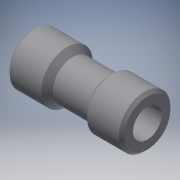
# Autodesk Inventor part: motor_coupling
Saved by Autodesk Inventor 2016 (Build 200138000, 138)
## iProperties
Created: 2016-12-23
Part Number: motor_coupling
Material: Generic
Document SubType Name: Modeling
Designer: inorn
Density: 1 g/cm^3
Appearance: Brass - Satin
Author: inorn
Autodesk Inventor part; units mm, degrees
ref_plane "YZ Plane" through (0, 0, 0) normal (1, 0, 0) x (0, 1, 0)
ref_plane "XZ Plane" through (0, 0, 0) normal (0, 1, 0) x (-1, 0, 0)
ref_plane "XY Plane" through (0, 0, 0) normal (0, 0, 1) x (1, 0, 0)
sketch "Sketch1" plane through (0, 0, 0) normal (1, 0, 0) x (0, 1, 0)
  circle A0 centre (0, 0) radius 4.5
  dimension "d0" = 9
  constraints: 1 centre point, 1 coincident
  measures "d0" diameter of A0
extrude "Extrusion1" add sketch "Sketch1" along normal blind 6
sketch "Sketch2" plane through (6, 0, 0) normal (1, 0, 0) x (0, 0, -1)
  circle A0 centre (0, 0) radius 3.5
  dimension "d3" = 7
  constraints: 1 centre point, 1 coincident
  measures "d3" diameter of A0
extrude "Extrusion2" add sketch "Sketch2" along normal blind 8
sketch "Sketch3" plane through (14, 0, 0) normal (1, 0, 0) x (0, 0, -1)
  circle A0 centre (0, 0) radius 4.5 projected
extrude "Extrusion3" add sketch "Sketch3" along normal blind 6
chamfer "Chamfer1" distance 1 angle 45 2 edges at (6, 0, 3.5) (14, 0, 3.5)
chamfer "Chamfer2" distance 0.5 angle 45 2 edges at (0, -4.5, 0) (20, 0, 4.5)
sketch "Sketch4" plane through (0, 0, 0) normal (-1, 0, 0) x (0, 0, 1)
  circle A0 centre (0, 0) radius 3.5 projected
  circle A1 centre (0, 0) radius 2.5
  dimension "d14" = 5
  constraints: 1 centre point, 1 coincident
  measures "d14" diameter of A1
extrude "Extrusion4" cut sketch "Sketch4" against normal through all contours A1
body "Solid1"
